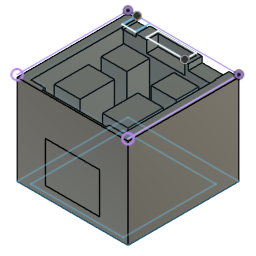
Aiwa (Autodesk Fusion 360 design; units mm, degrees)
part number: 2026-08-31-19-31-07-818
Autodesk Fusion 360 part; units mm, degrees
sketch "Sketch1" plane through (0, 0, 0) normal (0, 0, 1) x (1, 0, 0)
  line L0 (-50, 50) -> (50, 50)
  line L1 (50, 50) -> (50, -50)
  line L2 (50, -50) -> (-50, -50)
  line L3 (-50, -50) -> (-50, 50)
  line L4 (-60, 65) -> (60, 65)
  line L5 (60, 65) -> (60, -55)
  line L6 (60, -55) -> (-60, -55)
  line L7 (-60, -55) -> (-60, 65)
  dimension "d54" = 120
  dimension "d55" = 120
  dimension "d56" = 5
  constraint horizontal L0
  constraint vertical L1
  constraint horizontal L2
  constraint vertical L3
  constraint horizontal L4
  constraint vertical L5
  constraint horizontal L6
  constraint vertical L7
  measures "d54" distance of L4.start L6.end
  measures "d55" distance of L4.start L4.end
  measures "d56" distance of L2 L6
extrude "Extrude1" add sketch "Sketch1" along normal blind 5 contours L0 L1 L2 L3 makes body 1
extrude "Extrude2" add sketch "Sketch1" along normal blind 15 bodies 1
extrude "Extrude3" add 1 faces at (-16.6667, 60, 15) along direction (0, 0, 1) blind 85 on bodies 1 bodies 1
sketch "Sketch2" plane through (0, -55, 0) normal (0, -1, 0) x (1, 0, 0)
  line L0 (-60, 0) -> (60, 0)
  line L1 (60, 0) -> (60, 100)
  line L2 (60, 100) -> (-60, 100)
  line L3 (-60, 100) -> (-60, 0)
  line L4 (-29.25, 55.5) -> (29.25, 55.5)
  line L5 (29.25, 55.5) -> (29.25, 11.5)
  line L6 (29.25, 11.5) -> (-29.25, 11.5)
  line L7 (-29.25, 11.5) -> (-29.25, 55.5)
  line L8 (60, 0) -> (-60, 0)
  dimension "d7" = 58.5
  dimension "d8" = 44
  dimension "d9" = 30.75
  dimension "d10" = 30.75
  dimension "d11" = 11.5
  constraint horizontal L4
  constraint vertical L5
  constraint horizontal L6
  constraint vertical L7
  measures "d7" distance of L4.start L4.end
  measures "d8" distance of L4.start L6.end
  measures "d9" distance of L1 L5
  measures "d10" distance of L3 L7
  measures "d11" distance of L6 L8
surface "Extrude4" add extruded along (0, -1, 0) between 0 and -5 profiles "Sketch2" section 1 contours L4 L5 L6 L7 separate body makes body 2
surface "Extrude5" add extruded along (0, -1, 0) between 0 and -10 profiles "Sketch2" section 1 contours L4 L5 L6 L7 separate body makes body 3
sketch "Sketch3" plane through (0, -50, 0) normal (0, 1, 0) x (-1, 0, 0)
  line L0 (-50, 5) -> (50, 5)
  line L1 (50, 5) -> (50, 100)
  line L2 (50, 100) -> (-50, 100)
  line L3 (-50, 100) -> (-50, 5)
  line L4 (27.5, 61.5) -> (-27.5, 61.5)
  line L5 (-27.5, 61.5) -> (-27.5, 10)
  line L6 (-27.5, 10) -> (27.5, 10)
  line L7 (27.5, 10) -> (27.5, 61.5)
  line L8 (-29.25, 55.5) -> (-29.25, 11.5)
  line L9 (60, 100) -> (60, 0)
  line L10 (-60, 0) -> (-60, 100)
  line L11 (-60, 0) -> (60, 0)
  dimension "d16" = 55
  dimension "d17" = 51.5
  dimension "d20" = 32.5
  dimension "d21" = 32.5
  dimension "d22" = 10
  constraint horizontal L4
  constraint vertical L5
  constraint horizontal L6
  constraint vertical L7
  measures "d16" distance of L4.start L4.end
  measures "d17" distance of L4.start L6.end
  measures "d20" distance of L7 L9
  measures "d21" distance of L5 L10
  measures "d22" distance of L6 L11
sketch "Sketch4" plane through (0, 0, 100) normal (0, 0, 1) x (-1, 0, 0)
  line L0 (-50, 50) -> (50, 50)
  line L1 (50, 50) -> (50, -50)
  line L2 (50, -50) -> (-50, -50)
  line L3 (-50, -50) -> (-50, 50)
  line L4 (60, 55) -> (-60, 55)
  line L5 (-60, 55) -> (-60, -65)
  line L6 (-60, -65) -> (60, -65)
  line L7 (60, -65) -> (60, 55)
  line L8 (34.6, 49) -> (-34.6, 49)
  line L9 (-34.6, 49) -> (-34.6, 53)
  line L10 (-34.6, 53) -> (34.6, 53)
  line L11 (34.6, 53) -> (34.6, 49)
  line L12 (27.5, 50) -> (-27.5, 50)
  line L13 (-60, -65) -> (-60, 55)
  line L14 (60, 55) -> (60, -65)
  line L15 (29.25, 55) -> (-29.25, 55)
  dimension "d23" = 69.2
  dimension "d24" = 4
  dimension "d26" = 25.4
  dimension "d27" = 25.4
  dimension "d30" = 2
  constraint horizontal L8
  constraint vertical L9
  constraint horizontal L10
  constraint vertical L11
  measures "d23" distance of L8.start L8.end
  measures "d24" distance of L8 L10
  measures "d26" distance of L9 L13
  measures "d27" distance of L11 L14
  measures "d30" distance of L10 L15
extrude "Extrude6" add sketch "Sketch3" along normal blind 10 separate body contours L4 L5 L6 L7 makes body 4
extrude "Extrude7" cut sketch "Sketch4" against normal blind 8.5 contours L0 L8 L9 L11 L12 | L0 L9 L10 L11 L12 bodies 1
sketch "Sketch5" plane through (0, 0, 61.5) normal (0, 0, 1) x (-1, 0, 0)
  line L0 (27.5, 50) -> (-27.5, 50)
  line L1 (-27.5, 50) -> (-27.5, 40)
  line L2 (-27.5, 40) -> (27.5, 40)
  line L3 (27.5, 40) -> (27.5, 50)
  line L4 (27.5, 49) -> (-27.5, 49)
  line L5 (-27.5, 49) -> (-27.5, 50)
  line L6 (-27.5, 50) -> (27.5, 50)
  line L7 (27.5, 50) -> (27.5, 49)
  dimension "d33" = 1
  constraint horizontal L4
  constraint vertical L5
  constraint horizontal L6
  constraint vertical L7
  constraint coincident L0.end L1.start
  constraint coincident L3 L4.start
  measures "d33" distance of L4 L6
extrude "Extrude8" cut sketch "Sketch5" against normal blind 85 contours L0 L1 L3 L4 L5 L6 L7 bodies 4
extrude "Extrude9" cut 1 faces at (11.5333, -52, 91.5) along direction (0, 0, -1) blind 76.5 on bodies 1 bodies 1
sketch "Sketch6" plane through (0, 0, 5) normal (0, 0, 1) x (-1, 0, 0)
  line L0 (50, 50) -> (-50, 50)
  line L1 (-50, 50) -> (-50, -50)
  line L2 (-50, -50) -> (50, -50)
  line L3 (50, -50) -> (50, 50)
  line L4 (41.2638, -41.757) -> (13.4806, -41.757)
  line L5 (13.4806, -41.757) -> (13.4806, -17.2617)
  line L6 (13.4806, -17.2617) -> (41.2638, -17.2617)
  line L7 (41.2638, -17.2617) -> (41.2638, -41.757)
  line L8 (-12.823, -41.757) -> (-39.823, -41.757)
  line L9 (-39.823, -41.757) -> (-39.823, -17.2617)
  line L10 (-39.823, -17.2617) -> (-12.823, -17.2617)
  line L11 (-12.823, -17.2617) -> (-12.823, -41.757)
  line L12 (40.7706, -3.1236) -> (12.823, -3.1236)
  line L13 (12.823, -3.1236) -> (12.823, 34.0303)
  line L14 (12.823, 34.0303) -> (40.7706, 34.0303)
  line L15 (40.7706, 34.0303) -> (40.7706, -3.1236)
  line L16 (-12.4942, -3.1236) -> (-40, -3.1236)
  line L17 (-40, -3.1236) -> (-40, 35)
  line L18 (-40, 35) -> (-12.4942, 35)
  line L19 (-12.4942, 35) -> (-12.4942, -3.1236)
  dimension "d38" = 27
  constraint horizontal L4
  constraint vertical L5
  constraint horizontal L6
  constraint vertical L7
  constraint horizontal L8
  constraint vertical L9
  constraint horizontal L10
  constraint vertical L11
  constraint horizontal L12
  constraint vertical L13
  constraint horizontal L14
  constraint vertical L15
  constraint horizontal L16
  constraint vertical L17
  constraint horizontal L18
  constraint vertical L19
  measures "d38" distance of L8.start L8.end
extrude "Extrude10" add sketch "Sketch6" along normal blind 85 contours L4 L5 L6 L7 bodies 1
extrude "Extrude11" add sketch "Sketch6" along normal blind 85 contours L8 L9 L10 L11 bodies 1
extrude "Extrude12" add sketch "Sketch6" along normal blind 85 contours L16 L17 L18 L19 bodies 1
extrude "Extrude13" add sketch "Sketch6" along normal blind 85 contours L12 L13 L14 L15 bodies 1
sketch "Sketch7" plane through (0, 0, 100) normal (0, 0, 1) x (-1, 0, 0)
  line L0 (60, 55) -> (-60, 55)
  line L1 (-60, 55) -> (-60, -65)
  line L2 (-60, -65) -> (60, -65)
  line L3 (60, -65) -> (60, 55)
  line L4 (-34.6, 50) -> (-34.6, 53)
  line L5 (-34.6, 53) -> (34.6, 53)
  line L6 (34.6, 53) -> (34.6, 50)
  line L7 (34.6, 50) -> (50, 50)
  line L8 (50, 50) -> (50, -50)
  line L9 (50, -50) -> (-50, -50)
  line L10 (-50, -50) -> (-50, 50)
  line L11 (-50, 50) -> (-34.6, 50)
  line L12 (24.7747, -62.3889) -> (-16.4562, -62.3889)
  line L13 (-16.4562, -62.3889) -> (-16.4562, -50)
  line L14 (-16.4562, -50) -> (24.7747, -50)
  line L15 (24.7747, -50) -> (24.7747, -62.3889)
  line L16 (60, 55) -> (60, -65)
  line L17 (-60, -65) -> (-60, 55)
  line L18 (60, -65) -> (-60, -65)
  line L19 (50.2183, -65) -> (36.2183, -65)
  line L20 (36.2183, -65) -> (36.2183, -49)
  line L21 (36.2183, -49) -> (50.2183, -49)
  line L22 (50.2183, -49) -> (50.2183, -65)
  dimension "d57" = 35.2253
  dimension "d58" = 43.5438
  dimension "d59" = 2.6111
  dimension "d60" = 41.2309
  dimension "d61" = 12.3889
  dimension "d62" = 14
  dimension "d63" = 16
  constraint horizontal L12
  constraint vertical L13
  constraint horizontal L14
  constraint vertical L15
  constraint coincident L9 L13.end
  constraint horizontal L19
  constraint vertical L20
  constraint horizontal L21
  constraint vertical L22
  constraint coincident L2 L19.start
  measures "d57" distance of L15 L16
  measures "d58" distance of L13 L17
  measures "d59" distance of L12 L18
  measures "d60" distance of L12.start L12.end
  measures "d61" distance of L12.start L14.end
  measures "d62" distance of L19.start L19.end
  measures "d63" distance of L19.start L21.end
extrude "Extrude14" cut sketch "Sketch7" against normal blind 15 contours L9 L12 L13 L14 L15 bodies 1
extrude "Extrude15" cut 1 faces at (42.1521, 59.1296, 100) along direction (0, 0, -1) blind 5 on bodies 1 bodies 1
sketch "Sketch8" plane through (12.4942, 0, 0) normal (-1, 0, 0) x (0, -1, 0)
  line L0 (-3.1236, 5) -> (35, 5)
  line L1 (35, 5) -> (35, 90)
  line L2 (35, 90) -> (-3.1236, 90)
  line L3 (-3.1236, 90) -> (-3.1236, 5)
  line L4 (34.0303, 5) -> (-3.1236, 5)
  dimension "d51" = 85
  measures "d51" distance of L2 L4
extrude "Extrude16" add 1 faces at (42.1521, 59.1296, 95) along direction (0, 0, 1) blind 2.5 on bodies 1 bodies 1
extrude "Extrude17" cut sketch "Sketch7" against normal blind 5.5 contours L2 L8 L9 L18 L19 L20 L21 L22 bodies 1
sketch "Sketch9" plane through (0, 0, 100) normal (0, 0, 1) x (-1, 0, 0)
  line L0 (-20.206, -65) -> (-49.206, -65)
  line L1 (-49.206, -65) -> (-49.206, -49.2281)
  line L2 (-49.206, -49.2281) -> (-20.206, -49.2281)
  line L3 (-20.206, -49.2281) -> (-20.206, -65)
  line L4 (-50, -50) -> (-50, 50)
  line L5 (-60, -65) -> (36.2183, -65)
  line L6 (60, -65) -> (-60, -65)
  dimension "d66" = 29
  dimension "d67" = 0.794
  dimension "d70" = 96.2183
  dimension "d71" = 120
  constraint horizontal L0
  constraint vertical L1
  constraint horizontal L2
  constraint vertical L3
  measures "d66" distance of L0.start L0.end
  measures "d67" distance of L1 L4
  measures "d70" distance of L5.start L5.end
  measures "d71" distance of L6.start L5.start
extrude "Extrude18" cut sketch "Sketch9" against normal blind 8.75 bodies 1
